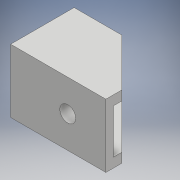
# Autodesk Inventor part: ブラケット
Saved by Autodesk Inventor 2017 (Build 210142000, 142)
## iProperties
Part Number: ブラケット
Material: 一般
Document SubType Name: Modeling
Designer: highs
Density: 1 g/cm^3
Appearance: 既定
Author: highs
Autodesk Inventor part; units mm, degrees
ref_plane "YZ Plane" through (0, 0, 0) normal (1, 0, 0) x (0, 1, 0)
ref_plane "XZ Plane" through (0, 0, 0) normal (0, 1, 0) x (-1, 0, 0)
ref_plane "XY Plane" through (0, 0, 0) normal (0, 0, 1) x (1, 0, 0)
sketch "スケッチ1" plane through (0, 0, 0) normal (0, 0, 1) x (1, 0, 0)
  line L0 (0, 0) -> (30, 0)
  line L1 (30, 0) -> (30, 5)
  line L2 (30, 5) -> (15, 20)
  line L3 (15, 20) -> (0, 20)
  line L4 (0, 20) -> (0, 0)
  dimension "d0" = 20
  dimension "d1" = 30
  dimension "d2" = 15
  dimension "d3" = 5
  constraints: 10 end point, 2 perpendicular, 1 horizontal, 1 parallel
  measures "d0" distance of L3.end L0.start
  measures "d1" distance of L0.start L0.end
  measures "d2" distance of L2.end L3.end
  measures "d3" distance of L0.end L1.end
extrude "押し出し1" add sketch "スケッチ1" along normal blind 20
sketch "スケッチ2" plane through (0, 20, 0) normal (0, 1, 0) x (1, 0, 0)
  line L0 (4.4, -3) -> (30, -3)
  line L1 (30, -3) -> (30, -17)
  line L2 (30, -17) -> (4.4, -17)
  line L3 (4.4, -17) -> (4.4, -3)
  line L4 (15, 0) -> (0, 0) projected
  line L5 (15, -20) -> (0, -20) projected
  line L6 (0, 0) -> (0, -20) projected
  line L7 (30, 0) -> (30, -20) projected
  dimension "d7" = 3
  dimension "d8" = 3
  dimension "d9" = 4.4
  constraints: 8 end point, 2 parallel, 1 horizontal, 1 perpendicular, 1 point on line
  measures "d7" distance between parallel lines of L4 L0
  measures "d8" distance between parallel lines of L5 L2
  measures "d9" distance between parallel lines of L3 L6
extrude "押し出し2" cut sketch "スケッチ2" against normal blind 15.6
chamfer "面取り1" distance 2 angle 45 2 edges at (4.4, 20, 10) (30, 4.4, 10)
sketch "スケッチ3" plane through (0, 0, 0) normal (-1, 0, 0) x (0, 0, 1)
  line L0 (0, 0) -> (20, 0) construction
  line L1 (10, 0) -> (10, 20) construction
  line L2 (0, 20) -> (20, 20) construction
  line L3 (0, 5) -> (0, 20) construction
  circle A0 centre (10, 10) radius 2.5
  dimension "d15" = 5
  constraints: 3 midpoint, 2 end point, 1 centre point
  measures "d15" diameter of A0
extrude "押し出し3" cut sketch "スケッチ3" against normal through all
sketch "スケッチ4" plane through (0, 0, 0) normal (0, -1, 0) x (1, 0, 0)
  line L0 (30, 0) -> (30, 20) construction
  line L1 (30, 10) -> (0, 10) construction
  circle A0 centre (18, 10) radius 2.5
  point P0 (0, 0)
  dimension "d18" = 5
  dimension "d19" = 12
  constraints: 2 end point, 1 centre point, 1 horizontal, 1 midpoint, 1 point on line
  measures "d18" diameter of A0
  measures "d19" distance from line of L0 A0.centre
extrude "押し出し4" cut sketch "スケッチ4" against normal up to next
